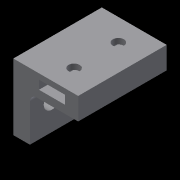
# Autodesk Inventor part: ExtruderTimingBeltHolder
Saved by Autodesk Inventor 2015 (Build 190159000, 159)
## iProperties
Created: 2014-11-14
Part Number: ExtruderTimingBeltHolder
Material: Generic
Document SubType Name: Modeling
Designer: Scott
Density: 1 g/cm^3
Appearance: Default
Author: Scott
Autodesk Inventor part; units mm, degrees
ref_plane "YZ Plane" through (0, 0, 0) normal (1, 0, 0) x (0, 1, 0)
ref_plane "XZ Plane" through (0, 0, 0) normal (0, 1, 0) x (-1, 0, 0)
ref_plane "XY Plane" through (0, 0, 0) normal (0, 0, 1) x (1, 0, 0)
sketch "Sketch1" plane through (0, 0, 0) normal (1, 0, 0) x (0, 1, 0)
  line L0 (0, 0) -> (15.24, 0)
  line L1 (15.24, 0) -> (15.24, -20.32)
  line L2 (15.24, -20.32) -> (0, -20.32)
  line L3 (0, -20.32) -> (0, 0)
  dimension "d0" = 15.24
  dimension "d1" = 20.32
  constraints: 8 end point, 3 perpendicular, 1 horizontal
  measures "d0" distance of L0.start L0.end
  measures "d1" distance of L0.end L1.end
extrude "Extrusion1" add sketch "Sketch1" along normal blind 3.81
sketch "Sketch2" plane through (0, 0, 0) normal (0, 0, 1) x (1, 0, 0)
  line L0 (3.81, 15.24) -> (8.89, 15.24)
  line L1 (8.89, 15.24) -> (14.89, 15.24)
  line L2 (14.89, 15.24) -> (14.89, 10.16)
  line L3 (14.89, 10.16) -> (3.81, 10.16)
  line L4 (3.81, 15.24) -> (3.81, 0) projected
  line L5 (8.89, 12.9701) -> (11.89, 12.9701)
  line L6 (11.89, 12.9701) -> (11.89, 11.9701)
  line L7 (11.89, 11.9701) -> (5.89, 11.9701)
  line L8 (5.89, 11.9701) -> (5.89, 12.9701)
  line L9 (5.89, 12.9701) -> (5.89, 13.9701)
  line L10 (5.89, 13.9701) -> (11.89, 13.9701)
  line L11 (11.89, 13.9701) -> (11.89, 12.9701)
  line L12 (3.81, 15.24) -> (3.81, 10.16)
  line L13 (0, 12.9701) -> (3.81, 12.9701)
  line L14 (5.89, 12.9701) -> (8.89, 12.9701)
  point P0 (0, 0)
  point P1 (0, 15.24)
  dimension "d4" = 8.89
  dimension "d5" = 6
  dimension "d6" = 5.08
  dimension "d7" = 8.89
  dimension "d8" = 3
  dimension "d9" = 1
  dimension "d10" = 6
  dimension "d11" = 1
  constraints: 28 end point, 6 perpendicular, 5 point on line, 4 horizontal, 1 collinear, 1 vertical
  measures "d4" distance of point (0, 15.24) L0.end
  measures "d5" distance of L0.end L1.end
  measures "d6" distance of L1.end L2.end
  measures "d7" distance of L13.start L5.start
  measures "d8" distance of L5.start L5.end
  measures "d9" distance of L5.end L6.end
  measures "d10" distance of L6.end L7.end
  measures "d11" distance of L8.end L9.end
extrude "Extrusion2" add sketch "Sketch2" against normal blind 20.32
sketch "Sketch3" plane through (5.89, 11.9701, 0) normal (0, 1, 0) x (1, 0, 0)
  line L0 (0, 0) -> (0, 5.08)
  line L1 (0, 0) -> (0, 20.32) projected
  line L2 (0, 5.08) -> (2.9845, 5.08)
  line L3 (6, 0) -> (6, 20.32) projected
  circle A0 centre (2.9845, 5.08) radius 1.27
  line L4 (-2.08, 0) -> (-2.08, 10.16)
  line L5 (-2.08, 0) -> (-2.08, 20.32) projected
  line L6 (-2.08, 10.16) -> (2.0052, 10.16)
  circle A1 centre (2.9845, 15.24) radius 1.27
  point P0 (-5.89, 0)
  dimension "d14" = 5.08
  dimension "d15" = 2.9845
  dimension "d16" = 2.54
  dimension "d17" = 10.16
  constraints: 8 end point, 2 centre point, 2 perpendicular, 1 coincident, 1 midpoint, 1 point on line, 1 symmetric about line, 1 other
  measures "d14" distance of L0.start L0.end
  measures "d15" distance of L0.end L2.end
  measures "d16" diameter of A0
  measures "d17" distance of L4.start L4.end
extrude "Extrusion3" cut sketch "Sketch3" along normal mid plane 20.32
sketch "Sketch4" plane through (3.81, 0, 0) normal (1, 0, 0) x (0, 0, -1)
  line L0 (0, 0) -> (0, 6.35)
  line L1 (0, 10.16) -> (0, 0) projected
  line L2 (0, 6.35) -> (5.08, 6.35)
  circle A0 centre (5.08, 6.35) radius 1.905
  line L3 (0, 0) -> (10.16, 0)
  line L4 (0, 0) -> (20.32, 0) projected
  line L5 (10.16, 0) -> (10.16, 4.445)
  circle A1 centre (15.24, 6.35) radius 1.905
  dimension "d20" = 6.35
  dimension "d21" = 5.08
  dimension "d22" = 3.81
  dimension "d23" = 10.16
  constraints: 8 end point, 2 centre point, 1 coincident, 1 horizontal, 1 midpoint, 1 perpendicular, 1 point on line, 1 symmetric about line, 1 other
  measures "d20" distance of L0.start L0.end
  measures "d21" distance of L0.end L2.end
  measures "d22" diameter of A0
  measures "d23" distance of L0.start L3.end
extrude "Extrusion4" cut sketch "Sketch4" against normal blind 20.32
fillet "Fillet1" radius 1.5875 1 edges at (3.81, 10.16, -10.16)
body "Solid1"
